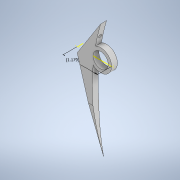
# Autodesk Inventor part: legV2
Saved by Autodesk Inventor 2022 (Build 260153000, 153)
## iProperties
Created: 2022-01-24
Part Number: legV2
Material: Generic
Document SubType Name: Modeling
Designer: money
Density: 1 g/cm^3
Appearance: Default
Author: money
Autodesk Inventor part; units mm, degrees
ref_plane "YZ Plane" through (0, 0, 0) normal (1, 0, 0) x (0, 1, 0)
ref_plane "XZ Plane" through (0, 0, 0) normal (0, 1, 0) x (-1, 0, 0)
ref_plane "XY Plane" through (0, 0, 0) normal (0, 0, 1) x (1, 0, 0)
sketch "Sketch1" plane through (0, 0, 0) normal (0, 0, 1) x (1, 0, 0)
  circle A0 centre (0, 0) radius 6.604
  arc A1 (-6.5253, -6.9387) -> (-4.4452, 8.4241) centre (0, 0) ccw
  line L0 (0, 27.271) -> (-20.415, -4.6403)
  line L1 (-20.415, -4.6403) -> (0, -73.9689)
  arc A2 (0, 27.271) -> (-4.4452, 8.4241) centre (172.4432, -23.349) ccw
  arc A3 (-6.5253, -6.9387) -> (0, -73.9689) centre (172.4432, -23.349) ccw
  dimension "d0" = 13.208
  dimension "d1" = 19.05
  constraints: 7 point on circle, 4 centre point, 4 end point, 2 coincident
  measures "d0" diameter of A0
  measures "d1" diameter of A1
extrude "Extrusion1" add sketch "Sketch1" along normal blind 5.08
sketch "Sketch2" plane through (0, 0, 0) normal (1, 0, 0) x (0, 1, 0)
  line L0 (-73.9689, 0) -> (-73.9689, 5.08) projected
  line L1 (-73.9689, 2.54) -> (-0.7706, 7.6585)
  line L2 (-0.7706, 7.6585) -> (-0.7706, -2.5785)
  line L3 (-0.7706, -2.5785) -> (-73.9689, 2.54)
  line L4 (-0.7706, -2.5785) -> (-76.3846, -2.5785)
  line L5 (-76.3846, -2.5785) -> (-76.3846, 10.5273)
  line L6 (-76.3846, 10.5273) -> (-0.7706, 10.5273)
  line L7 (-0.7706, 10.5273) -> (-0.7706, 7.6585)
  point P0 (0, 0)
  dimension "d4" = 86
  dimension "d5" = 86
  constraints: 14 end point, 2 perpendicular, 1 horizontal, 1 midpoint, 1 parallel, 1 point on line, 1 vertical
  measures "d4" angle of L1 L2
  measures "d5" angle of L3 L2
extrude "Extrusion2" cut sketch "Sketch2" against normal blind 25.7175 contours L3 L4 L5 L6 L7 L1
sketch "Sketch3" plane through (0, 0, 0) normal (1, 0, 0) x (0, 1, 0)
  line L0 (8.4241, 0) -> (27.271, 0) projected
  line L1 (15.3537, 0) -> (15.3537, 5.0379)
  circle A0 centre (15.3537, 2.519) radius 1.27
  point P0 (0, 0)
  dimension "d8" = 2.54
  constraints: 2 end point, 1 centre point, 1 midpoint, 1 perpendicular, 1 point on line
  measures "d8" diameter of A0
extrude "Extrusion3" cut sketch "Sketch3" against normal blind 25.7175
sketch "Sketch4" plane through (0, 0, 0) normal (0, 1, 0) x (-1, 0, 0)
  line L0 (20.415, 0) -> (20.415, 5.08) projected
  line L1 (6.5253, 5.08) -> (-9.525, 5.08) projected
  point P0 (0, 0)
  point P1 (4.4452, 5.08)
  dimension "d11" = 29.94
  measures "d11" distance of L0.end L1.end
body "Solid1"
